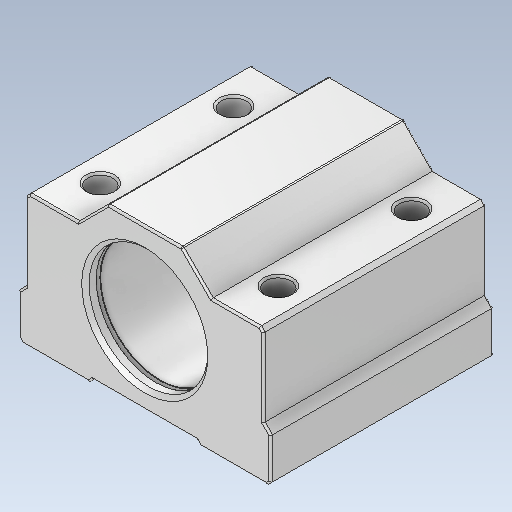
# Autodesk Inventor part: SC8UU body
Saved by Autodesk Inventor 2020.2 (Build 242310000, 310)
## iProperties
Created: 2020-07-09
Part Number: SC8UU body
Material: Ogólny
Document SubType Name: Modeling
Designer: Artur Lenart
Density: 1 g/cm^3
Appearance: Aluminium — polerowane
Mass: 12.2479 g
Surface Area: 64.4758 cm^2
Volume: 12.2479 cm^3
Author: Artur Lenart
Autodesk Inventor part; units mm, degrees
ref_plane "YZ Plane" through (0, 0, 0) normal (1, 0, 0) x (0, 1, 0)
ref_plane "XZ Plane" through (0, 0, 0) normal (0, 1, 0) x (-1, 0, 0)
sketch "Szkic1" plane through (0, 0, 0) normal (1, 0, 0) x (0, 1, 0)
  line L0 (0.5, 0) -> (6, 0)
  line L1 (22, 0) -> (22, -12) construction
  line L2 (22, -34) -> (18, -34) construction
  line L3 (0, -17) -> (11, -17) construction
  circle A0 centre (11, -17) radius 8
  line L4 (18, 0) -> (18, -1) construction
  line L5 (22, -12) -> (18, -8)
  line L6 (22, -12) -> (29.1229, -12) construction
  line L7 (22, -22) -> (18, -26)
  line L8 (22, -22) -> (32.7221, -22) construction
  line L9 (6, 0) -> (7, -1)
  line L10 (6, 0) -> (7.9702, 0) construction
  line L11 (7, -1) -> (17.5, -1)
  line L12 (6, 0) -> (22, 0) construction
  line L13 (18, -1.5) -> (18, -8)
  line L14 (22, -12) -> (22, -22)
  line L15 (22, -22) -> (22, -34) construction
  line L16 (18, -26) -> (18, -32.5)
  line L17 (18, -34) -> (6, -34) construction
  line L18 (17.5, -1) -> (18, -1.5)
  line L19 (17.3756, -0.6779) -> (19.849, -0.6779) construction
  line L20 (6, -34) -> (7, -33)
  line L21 (6, -34) -> (7.9702, -34) construction
  line L22 (17.5, -33) -> (18, -32.5)
  line L23 (7, -33) -> (17.5, -33)
  line L24 (6, -34) -> (0.5, -34)
  line L25 (18, -32.5) -> (18, -33)
  line L26 (0.5, 0) -> (0, -0.5)
  line L27 (0.5, -34) -> (0, -33.5)
  line L28 (0.5, -34) -> (0, -34) construction
  line L29 (0, -9.5) -> (0.5, -10)
  line L30 (0, -9.5) -> (3.9988, -9.5) construction
  line L31 (0.5, -10) -> (0.5, -24)
  line L32 (0, -24.5) -> (0.5, -24)
  line L33 (0, -34) -> (0, -24.5)
  line L34 (0, -9.5) -> (0, 0)
  line L35 (-6.5444, 0) -> (39.2665, 0) projected
  point P0 (17.3756, -33.3221)
  point P1 (3.25, 0)
  point P2 (0, -33.5)
  dimension "d0" = 22
  dimension "d1" = 34
  dimension "d3" = 16
  dimension "d5" = 135
  dimension "d6" = 135
  dimension "d7" = 10
  dimension "d8" = 12
  dimension "d9" = 45
  dimension "d12" = 45
  dimension "d13" = 0.5
  dimension "d15" = 0.5
  dimension "d16" = 45
  dimension "d17" = 10
  dimension "d19" = 11
  dimension "d20" = 0.5
  dimension "d21" = 18
  dimension "d22" = 135
  dimension "d23" = 1
  dimension "d24" = 6
  constraints: 70 end point, 26 perpendicular, 14 parallel, 11 symmetric about line, 9 horizontal, 9 point on line, 1 centre point, 1 coincident, 1 midpoint, 1 vertical, 2 other
  measures "d0" distance of L2.start L28.end
  measures "d1" distance of L1.start L2.start
  measures "d3" diameter of A0
  measures "d5" angle of L6 L5
  measures "d6" angle of L7 L8
  measures "d7" distance of L7.start L1.end
  measures "d8" distance of L1.start L1.end
  measures "d9" angle of L9 L10
  measures "d12" angle of L18 L19
  measures "d13" distance from line of L13.start L11
  measures "d15" distance of L26.end L34.end
  measures "d16" angle of L29 L30
  measures "d17" distance from line of L29.end L0
  measures "d19" distance from line of L34 L3.end
  measures "d20" distance between parallel lines of L34 L31
  measures "d21" distance between parallel lines of L34 L13
  measures "d22" angle of L26 L0
  measures "d23" distance between parallel lines of L11 L0
  measures "d24" distance from line of L0.end L34
extrude "Wyciągnięcie proste1" add sketch "Szkic1" along normal blind 30 contours L0 L9 L11 L18 L13 L5 L14 L7 L16 L22 L23 L20 L24 L27 L33 L32 L31 L29 L34 L26
chamfer "Faza1" distance 0.5 angle 45 2 edges at (30, 3, -17) (0, 3, -17)
ref_plane "Płaszczyzna konstrukcyjna1" through (0, 0.5, -17) normal (0, 0, -1) x (-1, 0, 0)
sketch "Szkic2" plane through (0, 0.5, -17) normal (0, 0, -1) x (-1, 0, 0)
  line L0 (-29.5, 18.5) -> (-0.5, 18.5) projected
  line L1 (-30, 21.5) -> (-30, 17.5) projected
  line L2 (-28.5, 18.5) -> (-28, 18.5)
  line L3 (-28, 18.5) -> (-28, 19.5)
  line L4 (-28, 19.5) -> (-28.5, 19.5)
  line L5 (-28.5, 19.5) -> (-28.5, 18.5)
  line L6 (0, 21.5) -> (-30, 21.5) projected
  line L7 (-15, 21.5) -> (-15, 18.5) construction
  line L8 (-1.5, 18.5) -> (-2, 18.5)
  line L9 (-2, 18.5) -> (-2, 19.5)
  line L10 (-2, 19.5) -> (-1.5, 19.5)
  line L11 (-1.5, 19.5) -> (-1.5, 18.5)
  line L12 (6, -0.5) -> (-36, -0.5) projected
  line L13 (-29.5, 2.5) -> (-29.5, 18.5) projected
  line L14 (-29.5, 10.5) -> (-0.5, 10.5) construction
  line L15 (-0.5, 18.5) -> (-0.5, 2.5) projected
  point P0 (0, -0.5)
  point P1 (-28.25, 18.5)
  point P2 (-1.75, 18.5)
  dimension "d31" = 0.5
  dimension "d32" = 1
  dimension "d33" = 1.5
  constraints: 20 end point, 5 midpoint, 5 symmetric about line, 2 parallel, 1 horizontal, 1 perpendicular, 1 point on line
  measures "d31" distance of L4.end L3.end
  measures "d32" distance of L3.end L2.end
  measures "d33" distance between parallel lines of L1 L5
revolve "Obrót1" cut sketch "Szkic2" angle 360 about axis through (29.5, 11, -17) along (-1, 0, 0)
sketch "Szkic3" plane through (0, 0, -33.5) normal (0, -1, 0) x (1, 0, 0)
  line L0 (24, 4.5) -> (6, 4.5) construction
  line L1 (6, 4.5) -> (6, 28.5) construction
  line L2 (6, 28.5) -> (24, 28.5) construction
  line L3 (24, 28.5) -> (24, 4.5) construction
  line L4 (0, 33.5) -> (30, 33.5) projected
  line L5 (0, 9) -> (0, 0) projected
  circle A0 centre (24, 4.5) radius 2
  circle A1 centre (6, 4.5) radius 2
  circle A2 centre (6, 28.5) radius 2
  circle A3 centre (24, 28.5) radius 2
  dimension "d35" = 18
  dimension "d36" = 24
  dimension "d37" = 5
  dimension "d38" = 6
  dimension "d39" = 4
  dimension "d40" = 4
  dimension "d41" = 4
  dimension "d42" = 4
  constraints: 8 end point, 4 centre point, 4 coincident, 2 parallel, 1 horizontal, 1 perpendicular
  measures "d35" distance of L1.end L2.end
  measures "d36" distance of L0.end L1.end
  measures "d37" distance between parallel lines of L4 L2
  measures "d38" distance between parallel lines of L5 L1
  measures "d39" diameter of A0
  measures "d40" diameter of A1
  measures "d41" diameter of A2
  measures "d42" diameter of A3
extrude "Wyciągnięcie proste2" cut sketch "Szkic3" against normal blind 8
sketch "Szkic4" plane through (24, 8, -5) normal (0, -1, 0) x (1, 0, 0)
  circle A0 centre (0, 0) radius 2 projected
  circle A1 centre (0, 0) radius 1.7
  circle A2 centre (-18, 0) radius 2 projected
  circle A3 centre (-18, 0) radius 1.7
  circle A4 centre (-18, -24) radius 2 projected
  circle A5 centre (-18, -24) radius 1.7
  circle A6 centre (0, -24) radius 2 projected
  circle A7 centre (0, -24) radius 1.7
  point P0 (-24, 5)
  dimension "d45" = 3.4
  dimension "d46" = 3.4
  dimension "d47" = 3.4
  dimension "d48" = 3.4
  constraints: 4 centre point, 4 coincident
  measures "d45" diameter of A1
  measures "d46" diameter of A3
  measures "d47" diameter of A5
  measures "d48" diameter of A7
extrude "Wyciągnięcie proste3" cut sketch "Szkic4" against normal up to surface (10 mm away) contours A1 | A3 | A5 | A7
chamfer "Faza2" distance 0.25 angle 45 8 edges at (22.3, 18, -29) (4.3, 18, -29) (4.3, 18, -5) (22.3, 18, -5) (22, 0, -5) (4, 0, -5) (22, 0, -29) (4, 0, -29)
fillet "Zaokrąglenie1" radius 0.25 42 edges at (0, 3.25, -34) (0, 0.25, -33.75) (0, 0, -29) (0, 0.25, -24.25) (0, 0.5, -17) (0, 0.25, -9.75) (0, 0, -5) (0, 0.25, -0.25) (0, 3.25, 0) (0, 6.5, -0.5) (0, 12.25, -1) (0, 17.75, -1.25) (0, 18, -4.75) (0, 20, -10) (0, 22, -17) (0, 20, -24) (0, 18, -29.25) (0, 17.75, -32.75) (0, 12.25, -33) (0, 6.5, -33.5) (30, 3.25, -34) (30, 6.5, -33.5) (30, 12.25, -33) (30, 17.75, -32.75) (30, 18, -29.25) (30, 20, -24) (30, 22, -17) (30, 20, -10) (30, 18, -4.75) (30, 17.75, -1.25) (30, 12.25, -1) (30, 6.5, -0.5) (30, 3.25, 0) (30, 0.25, -0.25) (30, 0, -5) (30, 0.25, -9.75) (30, 0.5, -17) (30, 0.25, -24.25) (30, 0, -29) (30, 0.25, -33.75) (15, 22, -22) (15, 22, -12)
chamfer "Faza3" distance 0.05 angle 45 4 edges at (2, 3, -17) (1.5, 3, -17) (28, 3, -17) (28.5, 3, -17)
